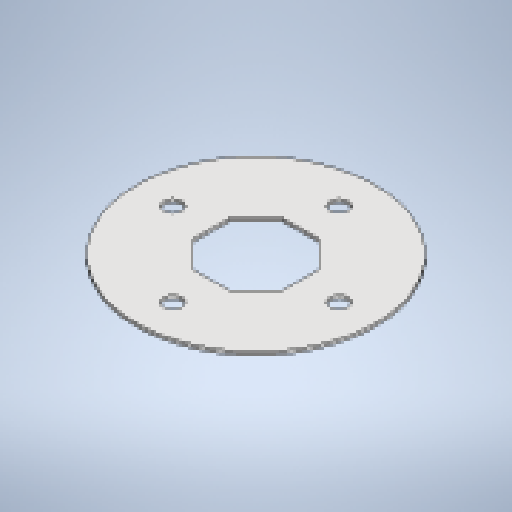
# Autodesk Inventor part: APN 1472  funnel FLANGE 1200 50-90
Saved by Autodesk Inventor 2025 (Build 290162010, 162A)
## iProperties
Created: 2025-06-24
Part Number: APN 1472  funnel FLANGE 1200 50-90
Material: Stainless Steel
Description: DIE16(5)|\ 90°|corrY -___°|X_____|bom___
Document SubType Name: Sheet Metal
Designer: user
Mass: 511.175 g
Surface Area: 458.858 cm^2
Volume: 63.8969 cm^3
Density: 8 g/cm^3
Flat Pattern Width: 23 cm
Flat Pattern Length: 23 cm
Flat Pattern Area: 529 cm^2
Sheet Metal Rule: Default
Sheet Metal Width: 230,000 mm
Sheet Metal Length: 230,000 mm
Sheet Metal Area: 52900,000 mm^2
Appearance: Default
Author: user
Autodesk Inventor part; units mm, degrees
ref_plane "YZ Plane" through (0, 0, 0) normal (1, 0, 0) x (0, 1, 0)
ref_plane "XZ Plane" through (0, 0, 0) normal (0, 1, 0) x (-1, 0, 0)
ref_plane "XY Plane" through (0, 0, 0) normal (0, 0, 1) x (1, 0, 0)
sketch "Sketch1" plane through (0, 0, 0) normal (0, 0, 1) x (1, 0, 0)
  circle A0 centre (0, 0) radius 115
  line L0 (55, 55) -> (-55, 55)
  line L1 (-55, 55) -> (-55, -55)
  line L2 (-55, -55) -> (55, -55)
  line L3 (55, -55) -> (55, 55)
  line L4 (55, 55) -> (-55, -55) construction
  line L5 (-55, 55) -> (55, -55) construction
  line L6 (-55, 22.7817) -> (-22.7817, 55)
  line L7 (22.7817, 55) -> (55, 22.7817)
  line L8 (55, -22.7817) -> (22.7817, -55)
  line L9 (-22.7817, -55) -> (-55, -22.7817)
  dimension "d157" = 230
  dimension "d158" = 110
  dimension "d159" = 110
  dimension "d171" = 110
  dimension "d172" = 110
  measures "d157" diameter of A0
  measures "d158" distance of L2.end L1.end
  measures "d159" distance of L1.end L0.end
  measures "d171" distance between parallel lines of L9 L7
  measures "d172" distance between parallel lines of L8 L6
extrude "Plate5" add sketch "Sketch1" along normal blind 3 contours A0 | L3 L7 L0 | L6 L1 L0 | L3 L2 L8 | L9 L2 L1
sketch "Sketch7" plane through (0, 0, 0) normal (0, 0, -1) x (-1, 0, 0)
  circle A0 centre (0, 90) radius 8.5
  circle A1 centre (0, 0) radius 90 construction
  dimension "d170" = 180
  dimension "d160" = 17
  constraints: 2 vertical alignment, 1 centre point, 1 coincident, 2 other
  measures "d160" diameter of A0
extrude "Cut1" cut sketch "Sketch7" against normal blind 3
pattern_circular "Circular Pattern1" count 4 over 360 about axis through (0, 0, -10) along (0, 0, 1) of "Cut1"
body "Solid3"
